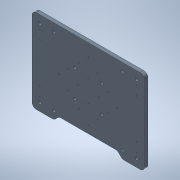
# Autodesk Inventor part: J010347
Saved by Autodesk Inventor 2020.3 (Build 243373000, 373)
## iProperties
RuleStatus: InUse
AfterDocSave0: file://Part Number Cleaner
Created: 2018-10-09
Material: ALUMINUM, 6061-T651
Vendor: HHMI: JRC - ID&F
Document SubType Name: Modeling
Designer: arnoldj
Density: 2.7 g/cm^3
Appearance: Steel Blue
Description: FLUGGER UPPER PLATE CYL
Project: COMMON
Part Number: J010347
LAB/DEPT: COMMON
REQUESTING SCIENTIST: COMMON
SURFACE ROUGHNESS: 63 Ra
DESIGN DEPARTMENT: HHMI: JRC - ID&F
SPECIAL FINISH: NONE
ALTERED ITEM PART NUMBER: N/A
ALTERED ITEM VENDOR: N/A
ALTERED ITEM DESCRIPTION: N/A
Author: arnoldj
Revision Number: -
Autodesk Inventor part; units mm, degrees
ref_plane "YZ Plane" through (0, 0, 0) normal (1, 0, 0) x (0, 1, 0)
ref_plane "XZ Plane" through (0, 0, 0) normal (0, 1, 0) x (-1, 0, 0)
ref_plane "XY Plane" through (0, 0, 0) normal (0, 0, 1) x (1, 0, 0)
sketch "Sketch1" plane through (0, 0, 0) normal (0, 0, 1) x (1, 0, 0)
  line L0 (0, 262.255) -> (0, -262.255) projected
  line L1 (-351.155, 0) -> (351.155, 0) projected
  line L2 (250.825, -187.325) -> (-250.825, -187.325)
  line L3 (-250.825, -187.325) -> (-250.825, 187.325)
  line L4 (-250.825, 187.325) -> (250.825, 187.325)
  line L5 (250.825, 187.325) -> (250.825, -187.325)
  line L6 (250.825, -187.325) -> (-250.825, 187.325) construction
  line L7 (-250.825, -187.325) -> (250.825, 187.325) construction
  line L8 (215.9, -152.4) -> (-215.9, -152.4) construction
  line L9 (-215.9, -152.4) -> (-215.9, 152.4) construction
  line L10 (-215.9, 152.4) -> (215.9, 152.4) construction
  line L11 (215.9, 152.4) -> (215.9, -152.4) construction
  line L12 (215.9, -152.4) -> (-215.9, 152.4) construction
  line L13 (-215.9, -152.4) -> (215.9, 152.4) construction
  line L14 (139.7, -139.7) -> (-139.7, -139.7) construction
  line L15 (-139.7, -139.7) -> (-139.7, 139.7) construction
  line L16 (-139.7, 139.7) -> (139.7, 139.7) construction
  line L17 (139.7, 139.7) -> (139.7, -139.7) construction
  line L18 (139.7, -139.7) -> (-139.7, 139.7) construction
  line L19 (-139.7, -139.7) -> (139.7, 139.7) construction
  line L20 (152.4, -165.1) -> (-152.4, -165.1)
  line L21 (-152.4, -165.1) -> (-152.4, -187.325)
  line L22 (-152.4, -187.325) -> (152.4, -187.325)
  line L23 (152.4, -187.325) -> (152.4, -165.1)
  line L24 (152.4, -165.1) -> (-152.4, -187.325) construction
  line L25 (-152.4, -165.1) -> (152.4, -187.325) construction
  line L26 (-64.7446, -24.1554) -> (-113.0554, -24.1554) construction
  line L27 (-113.0554, -24.1554) -> (-113.0554, 24.1554) construction
  line L28 (-113.0554, 24.1554) -> (-64.7446, 24.1554) construction
  line L29 (-64.7446, 24.1554) -> (-64.7446, -24.1554) construction
  line L30 (-64.7446, -24.1554) -> (-113.0554, 24.1554) construction
  line L31 (-113.0554, -24.1554) -> (-64.7446, 24.1554) construction
  line L32 (64.7446, -24.1554) -> (113.0554, -24.1554) construction
  line L33 (113.0554, -24.1554) -> (113.0554, 24.1554) construction
  line L34 (113.0554, 24.1554) -> (64.7446, 24.1554) construction
  line L35 (64.7446, 24.1554) -> (64.7446, -24.1554) construction
  line L36 (64.7446, -24.1554) -> (113.0554, 24.1554) construction
  line L37 (113.0554, -24.1554) -> (64.7446, 24.1554) construction
  circle A0 centre (-88.9, 0) radius 34.1609 construction
  circle A1 centre (88.9, 0) radius 34.1609 construction
  circle A2 centre (-88.9, 0) radius 41.275 construction
  circle A3 centre (88.9, 0) radius 41.275 construction
  circle A4 centre (0, 88.9) radius 41.275 construction
  circle A5 centre (0, -88.9) radius 41.275 construction
  line L38 (0, 130.175) -> (215.9, 130.175) construction
  line L39 (41.275, 88.9) -> (215.9, 88.9) construction
  point P0 (0, 0)
  point P1 (0, 0)
  point P2 (-139.7, 139.7)
  point P3 (-215.9, 152.4)
  point P4 (215.9, 152.4)
  point P5 (0, -176.2125)
  point P6 (-130.175, 0)
  point P7 (-47.625, 0)
  point P8 (-88.9, 41.275)
  point P9 (-88.9, -41.275)
  point P10 (47.625, 0)
  point P11 (130.175, 0)
  point P12 (88.9, 41.275)
  point P13 (88.9, -41.275)
  point P14 (-41.275, 88.9)
  point P15 (0, 47.625)
  point P16 (0, -47.625)
  point P17 (-41.275, -88.9)
  point P18 (0, -130.175)
  point P19 (41.275, -88.9)
  point P20 (215.9, -88.9)
  point P21 (215.9, -130.175)
  point P22 (-215.9, 130.175)
  point P23 (-215.9, 88.9)
  point P24 (-215.9, -88.9)
  point P25 (-215.9, -130.175)
  dimension "d0" = 501.65
  dimension "d1" = 374.65
  dimension "d2" = 431.8
  dimension "d3" = 304.8
  dimension "d4" = 279.4
  dimension "d5" = 279.4
  dimension "d17" = 0
  dimension "d18" = 0
  dimension "d28" = 0
  dimension "d29" = 22.225
  dimension "d30" = 304.8
  dimension "d36" = 88.9
  dimension "d37" = 88.9
  dimension "d38" = 48.3108
  dimension "d57" = 82.55
  dimension "d58" = 88.9
  dimension "d59" = 88.9
  dimension "d60" = 57.15
  dimension "d61" = 98.425
  dimension "d62" = 292.1
  dimension "d63" = 250.825
  dimension "d64" = 82.55
  constraints: 76 end point, 22 coincident, 16 point on circle, 12 midpoint, 12 parallel, 12 point on line, 8 perpendicular, 6 horizontal, 6 horizontal alignment, 4 centre point, 3 equal radius, 2 equal length, 22 other
  measures "d0" distance of L3.end L4.end
  measures "d1" distance of L2.end L3.end
  measures "d2" distance of L9.end L10.end
  measures "d3" distance of L8.end L9.end
  measures "d4" distance of L15.end L16.end
  measures "d5" distance of L14.end L15.end
  measures "d17" distance from line of L9 point (-215.9, 152.4)
  measures "d18" distance of point (215.9, 152.4) point (215.9, 152.4)
  measures "d29" distance of L20.end L21.end
  measures "d30" distance of L20.start L20.end
  measures "d38" distance of L27.end L28.end
  measures "d57" diameter of A2
  measures "d60" distance from line of L4 L38.start
  measures "d61" distance from line of A4.end L4
  measures "d62" distance from line of A4.end L5
  measures "d63" distance from line of L5 L38.start
  measures "d64" diameter of A4
extrude "Extrusion1" add sketch "Sketch1" against normal blind 15.875
hole "Hole1" at (215.9, -152.4, 0) at (-215.9, -152.4, 0) at (-215.9, 152.4, 0) at (215.9, 152.4, 0) direction (0, 0, -1) diameter 13.9954 end through all clearance for "Socket Head Cap Screw" size "M12" standard "Ansi Metric M Profile"
extrude "Extrusion2" cut sketch "Sketch1" against normal up to next contours L20 L23 L2 L0 | L0 L2 L21 L20
chamfer "Chamfer1" distance 22.225 angle 45 2 edges at (-152.4, -165.1, -7.9375) (152.4, -165.1, -7.9375)
fillet "Fillet1" radius 19.05 14 edges at (-250.825, -187.325, -7.9375) (250.825, -187.325, -7.9375) (250.825, 187.325, -7.9375) (-250.825, 187.325, -7.9375) (-152.4, -187.325, 0) (-152.4, -187.3249, -7.9375) (-152.4, -187.325, -7.9375) (-152.4, -187.325, -15.875) (152.4, -187.325, 0) (152.4, -187.3249, -7.9375) (152.4, -187.325, -7.9375) (152.4, -187.325, -15.875) (130.1751, -165.1, -7.9375) (-130.1751, -165.1, -7.9375)
hole "Hole3" at (-215.9, 152.4, 0) at (215.9, 152.4, 0) at (-130.175, 0, 0) at (-88.9, 41.275, 0) at (-47.625, 0, 0) at (-88.9, -41.275, 0) at (88.9, -41.275, 0) at (130.175, 0, 0) at (47.625, 0, 0) at (88.9, 41.275, 0) at (-41.275, 88.9, 0) at (0, 130.175, 0) at (41.275, 88.9, 0) at (0, 47.625, 0) at (-41.275, -88.9, 0) at (0, -47.625, 0) at (41.275, -88.9, 0) at (0, -130.175, 0) at (-215.9, 88.9, 0) at (-215.9, 130.175, 0) at (215.9, 130.175, 0) at (215.9, 88.9, 0) at (215.9, -88.9, 0) at (215.9, -130.175, 0) at (-215.9, -130.175, 0) at (-215.9, -88.9, 0) direction (0, 0, -1) diameter 4.134 end through all thread size "M5x0.8" class "6H" standard "ANSI Metric M Profile"
sketch "Sketch3" plane through (0, 0, 0) normal (0, 0, 1) x (1, 0, 0)
  line L0 (0, 213.36) -> (0, -213.36) projected
  line L1 (-213.36, 0) -> (213.36, 0) projected
  line L2 (152.4, -152.4) -> (-152.4, -152.4) construction
  line L3 (-152.4, -152.4) -> (-152.4, 152.4) construction
  line L4 (-152.4, 152.4) -> (152.4, 152.4) construction
  line L5 (152.4, 152.4) -> (152.4, -152.4) construction
  line L6 (152.4, -152.4) -> (-152.4, 152.4) construction
  line L7 (-152.4, -152.4) -> (152.4, 152.4) construction
  line L8 (60.325, -60.325) -> (-60.325, -60.325) construction
  line L9 (-60.325, -60.325) -> (-60.325, 60.325) construction
  line L10 (-60.325, 60.325) -> (60.325, 60.325) construction
  line L11 (60.325, 60.325) -> (60.325, -60.325) construction
  line L12 (60.325, -60.325) -> (-60.325, 60.325) construction
  line L13 (-60.325, -60.325) -> (60.325, 60.325) construction
  point P0 (0, 0)
  dimension "d46" = 304.8
  dimension "d47" = 304.8
  dimension "d48" = 120.65
  dimension "d49" = 120.65
  constraints: 24 end point, 8 coincident, 4 midpoint, 4 parallel, 2 horizontal, 2 perpendicular
  measures "d46" distance of L3.end L4.end
  measures "d47" distance of L2.end L3.end
  measures "d48" distance of L9.end L10.end
  measures "d49" distance of L8.end L9.end
hole "Hole4" at (-152.4, 152.4, 0) at (-60.325, 60.325, 0) at (60.325, 60.325, 0) at (152.4, 152.4, 0) at (-60.325, -60.325, 0) at (60.325, -60.325, 0) at (-152.4, -152.4, 0) at (152.4, -152.4, 0) direction (0, 0, -1) diameter 12.7 end through all
equation "\"d33\" = d29"
body "Solid1"
